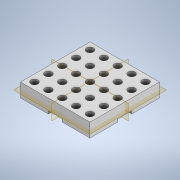
# Autodesk Inventor part: Tile
Saved by Autodesk Inventor 2022.4 (Build 264492010, 492A)
## iProperties
Created: 2025-02-20
Part Number: Tile
Material: Generic
Document SubType Name: Modeling
Designer: jan-m
Density: 1 g/cm^3
Appearance: Default
Author: jan-m
Autodesk Inventor part; units mm, degrees
sketch "Sketch1" plane through (0, 0, 0) normal (0, 1, 0) x (-1, 0, 0)
  line L0 (25, -25) -> (-25, -25)
  line L1 (-25, -25) -> (-25, 25)
  line L2 (-25, 25) -> (25, 25)
  line L3 (25, 25) -> (25, -25)
  line L4 (0, -35) -> (0, 35) projected
  line L5 (-35, 0) -> (35, 0) projected
  point P0 (0, 0)
  point P1 (0, -25)
  point P2 (25, 0)
  dimension "d0" = 50
  dimension "d1" = 50
  constraints: 8 end point, 2 midpoint, 2 parallel, 2 point on line, 1 horizontal, 1 perpendicular
  measures "d0" distance of L0.start L0.end
  measures "d1" distance of L2.end L0.start
extrude "Extrusion1" add sketch "Sketch1" along normal mid plane 10
sketch "Sketch2" plane through (0, -5, 0) normal (0, -1, 0) x (1, 0, 0)
  line L0 (-25, -25) -> (-25, 25) projected
  line L1 (-25, 5) -> (-17, 5)
  line L2 (-17, 5) -> (-17, -5)
  line L3 (-17, -5) -> (-25, -5)
  line L4 (-25, -5) -> (-25, 5)
  arc A0 (-17, -5) -> (-17, 5) centre (-17, 0) ccw
  line L5 (-35, 0) -> (35, 0) projected
  line L6 (-20, 5) -> (-20, -5)
  line L7 (0, -35) -> (0, 35) projected
  line L8 (-5, -25) -> (-5, -17)
  arc A1 (5, -17) -> (-5, -17) centre (0, -17) ccw
  line L9 (5, -17) -> (5, -25)
  line L10 (5, -25) -> (-5, -25)
  line L11 (-5, -20) -> (5, -20)
  line L12 (-5, -17) -> (5, -17)
  line L13 (25, -5) -> (17, -5)
  arc A2 (17, 5) -> (17, -5) centre (17, 0) ccw
  line L14 (17, 5) -> (25, 5)
  line L15 (25, 5) -> (25, -5)
  line L16 (20, -5) -> (20, 5)
  line L17 (17, -5) -> (17, 5)
  line L18 (5, 25) -> (5, 17)
  arc A3 (-5, 17) -> (5, 17) centre (0, 17) ccw
  line L19 (-5, 17) -> (-5, 25)
  line L20 (-5, 25) -> (5, 25)
  line L21 (5, 20) -> (-5, 20)
  line L22 (5, 17) -> (-5, 17)
  point P0 (0, 0)
  point P1 (-25, 0)
  point P2 (0, -25)
  point P3 (25, 0)
  point P4 (0, 25)
  dimension "d4" = 10
  dimension "d5" = 8
  dimension "d6" = 3
  dimension "d9" = 360
  constraints: 40 end point, 10 point on line, 8 point on circle, 4 centre point, 2 parallel, 2 perpendicular, 2 tangent, 1 horizontal, 1 midpoint, 57 other
  measures "d4" distance between parallel lines of L3 L1
  measures "d5" distance of L1.start L1.end
  measures "d6" distance between parallel lines of L2 L6
extrude "Extrusion2" cut sketch "Sketch2" against normal blind 2 contours L0 L5 L6 L3 | L0 L1 L6 L5 | L16 L14 L15 L5 | L5 L15 L13 L16 | L10 L8 L11 L7 | L7 L11 L9 L10 | L21 L19 L20 L7 | L7 L20 L18 L21
extrude "Extrusion3" cut sketch "Sketch2" against normal blind 4 contours L6 L5 L2 L3 | L6 L1 L2 L5 | L2 L5 A0 | L2 A0 L5 | A2 L17 L5 | L5 L17 A2 | L17 L14 L16 L5 | L5 L16 L13 L17 | L11 L8 L12 L7 | L7 L12 L9 L11 | L12 A1 L7 | L7 A1 L12 | A3 L22 L7 | L7 L22 A3 | L22 L19 L21 L7 | L7 L21 L18 L22
sketch "Sketch3" plane through (0, 5, 0) normal (0, 1, 0) x (1, 0, 0)
  circle A0 centre (-20, 20) radius 2.5
  line L0 (25, 25) -> (-25, 25) projected
  line L1 (-25, 25) -> (-25, -25) projected
  line L2 (-35, 0) -> (35, 0) projected
  line L3 (0, 35) -> (0, -35) projected
  circle A1 centre (-20, 10) radius 2.5
  circle A2 centre (-20, 0) radius 2.5
  circle A3 centre (-20, -10) radius 2.5
  circle A4 centre (-20, -20) radius 2.5
  circle A5 centre (-10, 20) radius 2.5
  circle A6 centre (-10, 10) radius 2.5
  circle A7 centre (-10, 0) radius 2.5
  circle A8 centre (-10, -10) radius 2.5
  circle A9 centre (-10, -20) radius 2.5
  circle A10 centre (0, 20) radius 2.5
  circle A11 centre (0, 10) radius 2.5
  circle A12 centre (0, 0) radius 2.5
  circle A13 centre (0, -10) radius 2.5
  circle A14 centre (0, -20) radius 2.5
  circle A15 centre (10, 20) radius 2.5
  circle A16 centre (10, 10) radius 2.5
  circle A17 centre (10, 0) radius 2.5
  circle A18 centre (10, -10) radius 2.5
  circle A19 centre (10, -20) radius 2.5
  circle A20 centre (20, 20) radius 2.5
  circle A21 centre (20, 10) radius 2.5
  circle A22 centre (20, 0) radius 2.5
  circle A23 centre (20, -10) radius 2.5
  circle A24 centre (20, -20) radius 2.5
  dimension "d15" = 5
  dimension "d16" = 5
  dimension "d17" = 5
  dimension "d20" = 10
  dimension "d23" = 10
  constraints: 25 centre point, 1 horizontal, 1 vertical, 48 other
  measures "d15" diameter of A0
  measures "d16" distance from line of L0 A0.centre
  measures "d17" distance from line of L1 A0.centre
  measures "d20" distance of A0.centre A1.centre
  measures "d23" distance of A0.centre A5.centre
extrude "Extrusion4" cut sketch "Sketch3" against normal blind 5 contours A0 | A10 L3 | L3 A10 | A2 L2 | L2 A2 | A11 L3 | L3 A11 | A7 L2 | L2 A7 | A12 L2 L3 | L3 L2 A12 | L3 A12 L2 | L2 A12 L3 | A17 L2 | L2 A17 | A22 L2 | L2 A22 | A13 L3 | L3 A13 | A14 L3 | L3 A14 | A1 | A3 | A4 | A5 | A6 | A8 | A9 | A15 | A16 | A18 | A19 | A20 | A21 | A23 | A24
body "Solid1"
